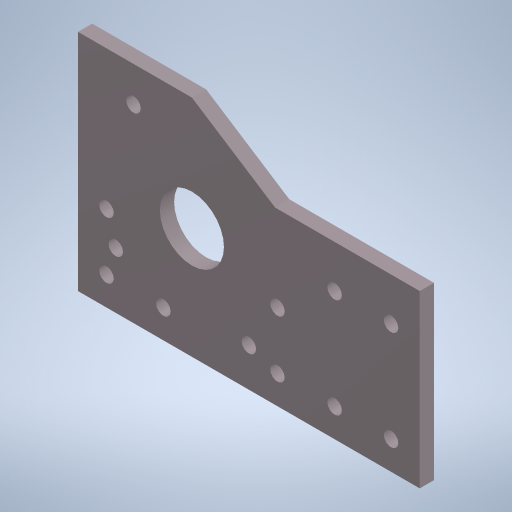
# Autodesk Inventor part: Y axis motor mount_before_change_31_03_2022
Saved by Autodesk Inventor 2023.2 (Build 272271000, 271)
## iProperties
Created: 2023-03-22
Part Number: Y axis motor mount_before_change_31_03_2022
Material: Aluminum 6061
Document SubType Name: Modeling
Designer: dmargari
Density: 2.7 g/cm^3
Appearance: Aluminum Cast
Author: dmargari
## iProperties of the stored document Y axis motor mount_3DPrint.ipt
Created: 2023-03-22
Part Number: Y axis motor mount_3DPrint
Material: Generic
Document SubType Name: Modeling
Designer: dmargari
Density: 1 g/cm^3
Appearance: Default
Author: dmargari
Autodesk Inventor part; units mm, degrees
ref_plane "YZ Plane" through (0, 0, 0) normal (1, 0, 0) x (0, 1, 0)
ref_plane "XZ Plane" through (0, 0, 0) normal (0, 1, 0) x (-1, 0, 0)
ref_plane "Work Plane1" through (0, 0, 0) normal (0, 0, 1) x (1, 0, 0)
sketch "Sketch1" plane through (0, 0, 0) normal (0, 0, 1) x (1, 0, 0)
  circle A0 centre (-83.6503, 950) radius 2.1 projected
  circle A1 centre (-83.6503, 970) radius 2.1 projected
  circle A2 centre (-63.6503, 950) radius 2.1 projected
  circle A3 centre (-43.6503, 950) radius 2.1 projected
  circle A4 centre (-23.6503, 950) radius 2.1 projected
  circle A5 centre (-23.6503, 970) radius 2.1 projected
  line L0 (-3.55, 0) -> (-3.55, 1000) projected
  line L1 (16.25, 0) -> (16.25, 1000) projected
  line L2 (-58.7503, 960) -> (-48.5503, 960) projected
  line L3 (-73.6503, 979.5) -> (-73.6503, 974.8314) projected
  line L4 (-78.7503, 980) -> (-74.1503, 980) projected
  line L5 (-33.6503, 974.8314) -> (-33.6503, 979.5) projected
  line L6 (-33.1503, 980) -> (-28.5503, 980) projected
  line L7 (-33.6503, 960) -> (-33.6503, 965.1685) projected
  line L8 (-38.7503, 960) -> (-33.6503, 960) projected
  line L9 (-73.6503, 960) -> (-68.5503, 960) projected
  line L10 (-73.6503, 965.1685) -> (-73.6503, 960) projected
  line L11 (-93.1503, 980) -> (-88.5503, 980) projected
  line L12 (-93.6503, 974.8314) -> (-93.6503, 979.5) projected
  line L13 (-93.6503, 960.207) -> (-93.6386, 965.287) projected
  line L14 (-93.6503, 954.8314) -> (-93.6503, 959.793) projected
  line L15 (-93.6503, 940.5) -> (-93.6503, 945.1685) projected
  line L16 (-88.4817, 940) -> (-93.1503, 940) projected
  line L17 (-14.1503, 940) -> (-18.8188, 940) projected
  circle A6 centre (-3.55, 950) radius 2.55
  circle A7 centre (16.25, 950) radius 2.55
  line L18 (26.35, 0) -> (26.35, 1000) projected
  line L19 (-14.1503, 940) -> (26.35, 940)
  line L20 (-14.1503, 940) -> (-93.1503, 940)
  line L21 (-33.6503, 960) -> (-33.7332, 960)
  line L22 (-14.15, 1000) -> (26.35, 1000)
  line L23 (26.35, 940) -> (26.35, 1000)
  line L24 (-33.6503, 960) -> (-33.6503, 960.1732)
  line L25 (-93.1503, 940) -> (-93.6503, 940)
  line L26 (-93.6503, 940) -> (-93.6503, 980)
  line L27 (-93.6503, 980) -> (-93.1503, 980)
  line L28 (-93.6503, 950) -> (27.9251, 950) construction
  circle A8 centre (-3.55, 985) radius 2.55
  circle A9 centre (16.25, 985) radius 2.55
  circle A10 centre (-80.3911, 959.775) radius 2.5
  circle A11 centre (-74.1633, 1006.5119) radius 2.5
  circle A12 centre (-33.6542, 953.5473) radius 2.5
  line L29 (-85.3287, 955.7671) -> (-21.9733, 1004.2234) construction
  line L30 (-29.4228, 948.3176) -> (-77.6558, 1011.3809) construction
  line L31 (-24.4599, 1000) -> (-14.15, 1000)
  line L32 (-93.6503, 980) -> (-93.6503, 1018.8249)
  line L33 (-93.6503, 1018.8249) -> (-53.65, 1018.8249)
  line L34 (-24.4599, 1000) -> (-53.65, 1018.8249)
  line L35 (-53.6502, 925.444) -> (-53.6503, 1034.9111) construction
  line L36 (-107.7091, 987) -> (-12.8224, 987) construction
  line L37 (-76.4503, 980) -> (8.1353, 980) construction
  line L38 (-33.6542, 953.5473) -> (-80.3911, 959.775) construction
  circle A13 centre (-53.6503, 980) radius 11.05
  circle A14 centre (-83.6503, 970) radius 2.55
  circle A15 centre (-83.6503, 950) radius 2.55
  circle A16 centre (-23.6503, 950) radius 2.55
  circle A17 centre (-63.6503, 950) radius 2.55
  circle A18 centre (-23.6503, 970) radius 2.55
  point P0 (0, 0)
  point P1 (-53.65, 970.886)
  point P2 (-93.65, 979.5)
  point P3 (-93.65, 974.8315)
  point P4 (-93.65, 959.793)
  point P5 (-93.65, 954.8315)
  point P6 (-93.65, 945.1686)
  point P7 (-93.65, 940.5)
  point P8 (-88.4815, 940)
  point P9 (-18.8186, 940)
  point P10 (-88.4816, 940)
  dimension "d0" = 5.1
  dimension "d2" = 5.1
  dimension "d9" = 5.1
  dimension "d10" = 15
  dimension "d11" = 15
  dimension "d17" = 47.15
  dimension "d22" = 5
  dimension "d23" = 5
  dimension "d24" = 5
  dimension "d29" = 20
  dimension "d30" = 7
  dimension "d31" = 47.15
  dimension "d32" = 22.1
  dimension "d33" = 5.1
  dimension "d34" = 5.1
  dimension "d35" = 5.1
  dimension "d36" = 5.1
  dimension "d37" = 5.1
  constraints: 40 end point, 13 centre point, 9 point on line, 6 coincident, 5 perpendicular, 3 horizontal, 2 collinear, 1 midpoint, 1 vertical, 4 other
  measures "d0" diameter of A6
  measures "d2" diameter of A7
  measures "d9" diameter of A9
  measures "d10" distance from line of L22 A8.centre
  measures "d11" distance from line of L22 A9.centre
  measures "d17" distance of A11.centre L38.end
  measures "d22" diameter of A12
  measures "d23" diameter of A10
  measures "d24" diameter of A11
  measures "d29" distance between parallel lines of L3 L35
  measures "d30" distance from line of L37.start L36
  measures "d31" distance of L38.start L38.end
  measures "d32" diameter of A13
  measures "d33" diameter of A14
  measures "d34" diameter of A15
  measures "d35" diameter of A16
  measures "d36" diameter of A17
  measures "d37" diameter of A18
extrude "Extrusion1" add sketch "Sketch1" along normal blind 5 contours A0 | A1 | A2 | A3 | A4 | A5 | L19 L17 L20 L16 L25 L26 L15 L14 L12 L32 L33 L34 L31 L22 L0 A8 A6 | L0 A6 A8 L22 L1 A9 A7 L19 | A6 L0 | L0 A6 | L1 A7 A9 L22 L18 L19 | A7 L1 | L1 A7 | A8 L0 | L0 A8 | A9 L1 | L1 A9 | A10 | A11 | A12 | A13 | A14 | A15 | A16 | A17 | A18
sketch "Sketch6" plane through (0, 0, 0) normal (0, 0, -1) x (-1, 0, 0)
  point P0 (0, 0)
  point P1 (83.6421, 950.0283)
  point P2 (63.6777, 949.9996)
  point P3 (23.6294, 949.9891)
  point P4 (3.544, 949.9934)
  point P5 (-16.2696, 949.986)
  point P6 (-16.2577, 984.9913)
  point P7 (3.5466, 984.9939)
  point P8 (74.1659, 1006.5019)
  point P9 (83.651, 970.0009)
  point P10 (80.4004, 959.774)
  point P11 (33.6669, 953.5674)
  point P12 (23.6003, 970.0426)
hole "Hole3" at (-83.6421, 950.0283, 0) at (-63.6777, 949.9996, 0) at (-23.6294, 949.9891, 0) at (-3.544, 949.9934, 0) at (16.2696, 949.986, 0) at (16.2577, 984.9913, 0) at (-3.5466, 984.9939, 0) at (-74.1659, 1006.5019, 0) at (-83.651, 970.0009, 0) at (-80.4004, 959.774, 0) at (-33.6669, 953.5674, 0) at (-23.6003, 970.0426, 0) direction (0, 0, 1) diameter 5.1 end through all
sketch "Sketch7" plane through (0, 0, 5) normal (0, 0, -1) x (-1, 0, 0)
  circle A0 centre (53.6503, 979) radius 4 projected
  circle A1 centre (53.6503, 979) radius 11.25
  point P0 (0, 0)
  dimension "d59" = 22.5
  constraints: 1 centre point, 1 coincident
  measures "d59" diameter of A1
extrude "Extrusion2" cut sketch "Sketch7" along normal blind 5 contours A0 | A1
body "Solid1"
